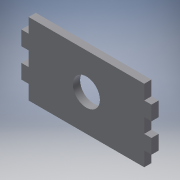
# Autodesk Inventor part: OctMiniSupport
Saved by Autodesk Inventor 2019 (Build 230136000, 136)
## iProperties
Created: 2019-01-14
Part Number: OctMiniSupport
Material: Wood (Birch)
Document SubType Name: Modeling
Designer: nxgam
Density: 0.55 g/cm^3
Appearance: Birch - Natural Polished
Author: nxgam
Autodesk Inventor part; units mm, degrees
ref_plane "YZ Plane" through (0, 0, 0) normal (1, 0, 0) x (0, 1, 0)
ref_plane "XZ Plane" through (0, 0, 0) normal (0, 1, 0) x (-1, 0, 0)
ref_plane "XY Plane" through (0, 0, 0) normal (0, 0, 1) x (1, 0, 0)
sketch "Sketch1" plane through (0, 0, 0) normal (0, 0, 1) x (1, 0, 0)
  line L0 (0, 0) -> (91.44, 0)
  line L1 (91.44, 0) -> (91.44, 50.8)
  line L2 (91.44, 50.8) -> (0, 50.8)
  line L3 (0, 50.8) -> (0, 0)
  line L4 (0, 50.8) -> (5.08, 50.8)
  line L5 (5.08, 50.8) -> (5.08, 40.64)
  line L6 (5.08, 40.64) -> (0, 40.64)
  line L7 (0, 40.64) -> (0, 50.8)
  line L8 (0, 30.48) -> (5.08, 30.48)
  line L9 (5.08, 30.48) -> (5.08, 20.32)
  line L10 (5.08, 20.32) -> (0, 20.32)
  line L11 (0, 20.32) -> (0, 30.48)
  line L12 (0, 10.16) -> (5.08, 10.16)
  line L13 (5.08, 10.16) -> (5.08, 0)
  line L14 (5.08, 0) -> (0, 0)
  line L15 (0, 0) -> (0, 10.16)
  line L16 (45.72, 50.8) -> (45.72, 0) construction
  line L17 (91.44, 50.8) -> (91.44, 0)
  line L18 (91.44, 50.8) -> (86.36, 50.8)
  line L19 (86.36, 50.8) -> (86.36, 40.64)
  line L20 (86.36, 40.64) -> (91.44, 40.64)
  line L21 (91.44, 40.64) -> (91.44, 50.8)
  line L22 (91.44, 30.48) -> (86.36, 30.48)
  line L23 (86.36, 30.48) -> (86.36, 20.32)
  line L24 (86.36, 20.32) -> (91.44, 20.32)
  line L25 (91.44, 20.32) -> (91.44, 30.48)
  line L26 (91.44, 10.16) -> (86.36, 10.16)
  line L27 (86.36, 10.16) -> (86.36, 0)
  line L28 (86.36, 0) -> (91.44, 0)
  line L29 (91.44, 0) -> (91.44, 10.16)
  dimension "d0" = 91.44
  dimension "d1" = 50.8
  dimension "d2" = 5.08
  dimension "d3" = 10.16
  dimension "d6" = 20.32
  constraints: 60 end point, 12 symmetric about line, 4 parallel, 2 horizontal, 2 midpoint, 2 perpendicular, 1 vertical, 16 other
  measures "d0" distance of L2.end L1.end
  measures "d1" distance of L1.end L0.end
  measures "d2" distance of L5.end L6.end
  measures "d3" distance of L4.end L5.end
  measures "d6" distance of L2.end L8.start
extrude "Extrusion1" add sketch "Sketch1" along normal blind 5.08 contours L13 L12 L3 L10 L9 L8 L6 L5 L2 L19 L20 L1 L22 L23 L24 L26 L27 L0
sketch "Sketch2" plane through (0, 0, 5.08) normal (0, 0, 1) x (1, 0, 0)
  line L0 (91.44, 20.32) -> (86.36, 20.32) projected
  line L1 (86.36, 20.32) -> (86.36, 30.48) projected
  line L2 (86.36, 30.48) -> (91.44, 30.48) projected
  line L3 (91.44, 30.48) -> (91.44, 40.64) projected
  line L4 (91.44, 40.64) -> (86.36, 40.64) projected
  line L5 (86.36, 40.64) -> (86.36, 50.8) projected
  line L6 (86.36, 50.8) -> (5.08, 50.8) projected
  line L7 (5.08, 50.8) -> (5.08, 40.64) projected
  line L8 (5.08, 40.64) -> (0, 40.64) projected
  line L9 (0, 40.64) -> (0, 30.48) projected
  line L10 (0, 30.48) -> (5.08, 30.48) projected
  line L11 (5.08, 30.48) -> (5.08, 20.32) projected
  line L12 (5.08, 20.32) -> (0, 20.32) projected
  line L13 (0, 20.32) -> (0, 10.16) projected
  line L14 (0, 10.16) -> (5.08, 10.16) projected
  line L15 (5.08, 10.16) -> (5.08, 0) projected
  line L16 (5.08, 0) -> (86.36, 0) projected
  line L17 (86.36, 0) -> (86.36, 10.16) projected
  line L18 (86.36, 10.16) -> (91.44, 10.16) projected
  line L19 (91.44, 10.16) -> (91.44, 20.32) projected
  line L20 (86.36, 50.8) -> (5.08, 50.8) construction
  line L21 (45.72, 50.8) -> (45.72, 0) construction
  line L22 (5.08, 0) -> (86.36, 0) construction
  line L23 (5.08, 25.4) -> (86.36, 25.4) construction
  circle A0 centre (45.72, 25.4) radius 9.525
  point P0 (0, 0)
  dimension "d13" = 19.05
  constraints: 5 midpoint, 4 end point, 1 centre point
  measures "d13" diameter of A0
extrude "Extrusion2" cut sketch "Sketch2" against normal blind 25.4 contours A0
equation "\"d6\" = 2 * d3"
body "Solid1"
